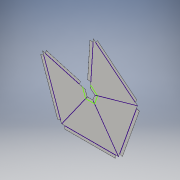
# Autodesk Inventor part: Nexus 7 3D hologram frame
Saved by Autodesk Inventor 2016 (Build 200138000, 138)
## iProperties
Created: 2017-08-31
Part Number: Nexus 7 3D hologram frame
Material: Generic
Document SubType Name: Modeling
Designer: student
Density: 1 g/cm^3
Appearance: Default
Author: student
Autodesk Inventor part; units mm, degrees
ref_plane "YZ Plane" through (0, 0, 0) normal (1, 0, 0) x (0, 1, 0)
ref_plane "XZ Plane" through (0, 0, 0) normal (0, 1, 0) x (-1, 0, 0)
ref_plane "XY Plane" through (0, 0, 0) normal (0, 0, 1) x (1, 0, 0)
sketch "Sketch1" plane through (0, 0, 0) normal (0, 0, 1) x (1, 0, 0)
  line L0 (-7.8362, 28.532) -> (7.1638, 28.532)
  line L1 (47.1638, -28.0341) -> (-47.8362, -28.0341)
  line L2 (7.1638, 28.532) -> (47.1638, -28.0341)
  line L3 (-7.8362, 28.532) -> (-47.8362, -28.0341)
  line L4 (-7.8362, 28.532) -> (-12.8438, 42.6835)
  line L5 (0.5011, 52.1252) -> (12.1714, 42.6835)
  line L6 (12.1714, 42.6835) -> (7.1638, 28.532)
  line L7 (-47.8362, -28.0341) -> (-79.5254, 61.5206)
  line L8 (-79.5254, 61.5206) -> (-12.8438, 42.6835)
  line L9 (47.1638, -28.0341) -> (78.853, 61.5206)
  line L10 (78.853, 61.5206) -> (12.1714, 42.6835)
  line L11 (78.853, 61.5206) -> (5.0003, 121.2702)
  line L12 (0.5011, 52.1252) -> (5.0003, 121.2702)
  point P0 (0, 0)
  point P1 (-0.3362, 28.532)
  point P2 (-0.3362, -28.0341)
  dimension "d0" = 69.28
  dimension "d1" = 95
  dimension "d2" = 15
  dimension "d3" = 56.566
  dimension "d4" = 69.28
  dimension "d16" = 15.0114
  dimension "d17" = 15.0114
  dimension "d18" = 15.0114
  dimension "d19" = 94.996
  dimension "d20" = 69.2912
  dimension "d21" = 94.996
  dimension "d22" = 69.2912
  dimension "d23" = 94.996
  dimension "d24" = 69.2912
  constraints: 26 end point, 4 parallel, 2 midpoint, 1 horizontal, 1 vertical alignment
  measures "d0" distance of L0.end L1.start
  measures "d1" distance of L1.start L1.end
  measures "d2" distance of L0.start L0.end
  measures "d3" distance between parallel lines of L1 L0
  measures "d4" distance of L0.start L1.end
  measures "d16" distance of L0.start L4.end
  measures "d17" distance of L5.end L0.end
  measures "d18" distance of L5.start L5.end
  measures "d19" distance of L1.end L7.end
  measures "d20" distance of L7.end L4.end
  measures "d21" distance of L1.start L9.end
  measures "d22" distance of L9.end L5.end
  measures "d23" distance of L9.end L11.end
  measures "d24" distance of L5.start L11.end
extrude "Extrusion2" add sketch "Sketch1" along normal blind 0.127
sketch "Sketch2" plane through (0, 0, 0.127) normal (0, 0, 1) x (1, 0, 0)
  line L0 (47.1638, -28.0341) -> (78.853, 61.5206) projected
  line L1 (53.6474, -24.9397) -> (81.9474, 55.0369)
  line L2 (78.0988, 68.6651) -> (12.1448, 122.0244)
  line L3 (5.0003, 121.2702) -> (0.5011, 52.1252) projected
  line L4 (-0.3988, 116.5308) -> (-4.2384, 57.5244)
  line L5 (-79.5254, 61.5206) -> (-47.8362, -28.0341) projected
  line L6 (-82.6198, 55.0369) -> (-54.3198, -24.9397)
  line L7 (-42.7562, -33.1141) -> (42.0838, -33.1141)
  line L8 (-7.8362, 28.532) -> (-12.8438, 42.6835) projected
  line L9 (-12.8438, 42.6835) -> (-79.5254, 61.5206) projected
  line L10 (78.853, 61.5206) -> (5.0003, 121.2702) projected
  line L11 (-4.2384, 57.5244) -> (0.8309, 57.1945)
  line L12 (-0.3988, 116.5308) -> (4.6704, 116.2009)
  line L13 (12.1448, 122.0244) -> (8.9496, 118.075)
  line L14 (78.0988, 68.6651) -> (74.9036, 64.7157)
  line L15 (78.853, 61.5206) -> (5.0003, 121.2702) projected
  line L16 (81.9474, 55.0369) -> (77.1584, 56.7315)
  line L17 (53.6474, -24.9397) -> (48.8584, -23.2451)
  line L18 (42.0838, -33.1141) -> (42.0838, -28.0341)
  line L19 (-47.8362, -28.0341) -> (47.1638, -28.0341) projected
  line L20 (-42.7562, -33.1141) -> (-42.7562, -28.0341)
  line L21 (-49.5308, -23.2451) -> (-54.3198, -24.9397)
  line L22 (-77.8307, 56.7315) -> (-82.6198, 55.0369)
  line L23 (-12.8438, 42.6835) -> (-79.5254, 61.5206) projected
  line L24 (-74.6367, 60.1395) -> (-73.2557, 65.0282)
  line L25 (-17.7328, 44.0646) -> (-16.414, 48.9705)
  line L26 (-73.2557, 65.0282) -> (-16.414, 48.9705)
  line L27 (-12.8438, 42.6835) -> (-8.3534, 41.4151)
  line L28 (-7.8362, 28.532) -> (-5.1428, 32.3417)
  line L29 (7.1638, 28.532) -> (-7.8362, 28.532) projected
  line L30 (-8.3534, 41.4151) -> (-5.1428, 32.3417)
  line L31 (12.1714, 42.6835) -> (7.1638, 28.532) projected
  line L32 (7.1638, 28.532) -> (4.4702, 32.342)
  line L33 (12.1714, 42.6835) -> (7.6811, 41.4151)
  line L34 (0.5011, 52.1252) -> (0.1988, 47.469)
  line L35 (0.5011, 52.1252) -> (12.1714, 42.6835) projected
  line L36 (0.1988, 47.469) -> (7.6811, 41.4151)
  line L37 (7.6811, 41.4151) -> (4.4702, 32.342)
  line L38 (4.4702, 32.342) -> (-5.1428, 32.3417)
  line L39 (8.9496, 118.075) -> (74.9036, 64.7157)
  point P0 (0, 0)
  dimension "d34" = 5.08
  dimension "d35" = 5.08
  dimension "d38" = 5.08
  dimension "d39" = 5.08
  dimension "d42" = 5.08
  dimension "d43" = 5.08
  dimension "d46" = 5.08
  dimension "d47" = 5.08
  dimension "d50" = 5.08
  dimension "d51" = 5.08
  dimension "d56" = 5.08
  dimension "d58" = 5.08
  dimension "d64" = 54.74
  dimension "d65" = 3.81
  dimension "d66" = 54.74
  dimension "d67" = 3.81
  dimension "d68" = 54.74
  dimension "d69" = 3.81
  dimension "d70" = 54.74
  dimension "d71" = 3.81
  dimension "d72" = 54.74
  dimension "d73" = 3.81
  dimension "d76" = 5.08
  constraints: 56 end point, 12 point on line, 8 perpendicular, 3 parallel, 1 collinear, 1 vertical
  measures "d34" distance of L4.start L12.end
  measures "d35" distance of L4.end L11.end
  measures "d38" distance of L2.end L13.end
  measures "d39" distance of L2.start L14.end
  measures "d42" distance of L1.end L16.end
  measures "d43" distance of L1.start L17.end
  measures "d46" distance of L7.start L20.end
  measures "d47" distance of L7.end L18.end
  measures "d50" distance of L22.start L6.start
  measures "d51" distance of L21.start L6.end
  measures "d56" distance of L24.start L24.end
  measures "d58" distance of L25.start L25.end
  measures "d64" angle of L8 L27
  measures "d65" distance from line of L8 L27.end
  measures "d66" angle of L29 L28
  measures "d67" distance from line of L8 L28.end
  measures "d68" angle of L29 L32
  measures "d69" distance from line of L29 L32.end
  measures "d70" angle of L31 L33
  measures "d71" distance from line of L31 L33.end
  measures "d72" angle of L35 L34
  measures "d73" distance from line of L35 L34.end
  measures "d76" distance from line of L3.start L12
extrude "Extrusion3" add sketch "Sketch2" against normal blind 0.127 contours L0 L16 L1 L17 | L18 L7 L20 L19 | L10 L13 L2 L14 | L21 L6 L22 L5 | L3 L11 L4 L12 | L24 L26 L25 L9 | L35 L33 L36 L34 | L27 L30 L28 L8 | L31 L32 L37 L33 | L28 L38 L32 L29
sketch "Sketch3" plane through (0, 0, 0.127) normal (0, 0, 1) x (1, 0, 0)
  line L0 (8.9496, 118.075) -> (74.9036, 64.7157)
  line L1 (78.853, 61.5206) -> (7.6811, 41.4151)
  line L2 (4.6704, 116.2009) -> (0.8309, 57.1945)
  line L3 (77.1584, 56.7315) -> (48.8584, -23.2451)
  line L4 (47.1638, -28.0341) -> (4.4702, 32.342)
  line L5 (42.0838, -28.0341) -> (-42.7562, -28.0341)
  line L6 (-5.1428, 32.3417) -> (-47.8362, -28.0341)
  line L7 (-49.5308, -23.2451) -> (-77.8307, 56.7315)
  line L8 (-74.6367, 60.1395) -> (-17.7328, 44.0646)
  line L9 (-12.8438, 42.6835) -> (-7.8364, 28.5324)
  line L10 (-7.8364, 28.5324) -> (7.164, 28.5324)
  line L11 (7.164, 28.5324) -> (12.1711, 42.6835)
  line L12 (12.1711, 42.6835) -> (0.5011, 52.1252)
  constraints: 26 end point, 3 point on line, 2 horizontal
body "Solid2"
